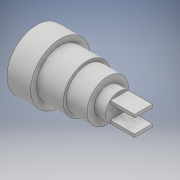
# Autodesk Inventor part: MJ-14
Saved by Autodesk Inventor 2017.3 (Build 213256000, 256)
## iProperties
Part Number: MJ-14
Material: 一般
Document SubType Name: Modeling
Designer: sktom
Density: 1 g/cm^3
Appearance: 既定
Author: sktom
Autodesk Inventor part; units mm, degrees
ref_plane "YZ Plane" through (0, 0, 0) normal (1, 0, 0) x (0, 1, 0)
ref_plane "XZ Plane" through (0, 0, 0) normal (0, 1, 0) x (-1, 0, 0)
ref_plane "XY Plane" through (0, 0, 0) normal (0, 0, 1) x (1, 0, 0)
sketch "スケッチ1" plane through (0, 0, 0) normal (0, 0, 1) x (1, 0, 0)
  line L0 (0, 0) -> (0, 5)
  line L1 (0, 5) -> (4, 5)
  line L2 (4, 5) -> (4, 4)
  line L3 (4, 4) -> (8.5, 4)
  line L4 (8.5, 4) -> (8.5, 3.5)
  line L5 (8.5, 3.5) -> (12, 3.5)
  line L6 (12, 3.5) -> (12, 2.25)
  line L7 (12, 2.25) -> (13.9, 2.25)
  line L8 (13.9, 2.25) -> (13.9, 0)
  line L9 (13.9, 0) -> (0, 0)
  dimension "d0" = 4
  dimension "d1" = 4.5
  dimension "d2" = 8
  dimension "d3" = 1.9
  dimension "d4" = 5
  dimension "d5" = 4
  dimension "d6" = 3.5
  dimension "d7" = 2.25
  constraints: 20 end point, 7 perpendicular, 2 horizontal, 1 vertical
  measures "d0" distance of L0.end L1.end
  measures "d1" distance of L2.end L3.end
  measures "d2" distance between parallel lines of L2 L6
  measures "d3" distance of L6.end L7.end
  measures "d4" distance of L0.start L0.end
  measures "d5" distance between parallel lines of L9 L3
  measures "d6" distance between parallel lines of L9 L5
  measures "d7" distance between parallel lines of L9 L7
revolve "回転1" add sketch "スケッチ1" angle 360 about axis through (13.9, 0, 0) along (-1, 0, 0)
sketch "スケッチ2" plane through (13.9, 0, 0) normal (1, 0, 0) x (0, 0, -1)
  circle A0 centre (0, 0) radius 2.25 projected
  line L0 (-1.6771, 1.5) -> (-1.1771, 1.5)
  line L1 (-1.1771, 1.5) -> (-1.1771, -1.5)
  line L2 (-1.1771, -1.5) -> (-1.6771, -1.5)
  line L3 (-1.6771, -1.5) -> (-1.6771, 1.5)
  line L4 (1.6771, 1.5) -> (1.1771, 1.5)
  line L5 (1.1771, 1.5) -> (1.1771, -1.5)
  line L6 (1.1771, -1.5) -> (1.6771, -1.5)
  line L7 (1.6771, -1.5) -> (1.6771, 1.5)
  point P0 (-1.1771, 0)
  point P1 (1.1771, 0)
  dimension "d9" = 3
  dimension "d10" = 0.5
  constraints: 16 end point, 4 parallel, 2 horizontal, 2 horizontal alignment, 2 midpoint, 2 perpendicular, 2 point on circle, 2 point on line, 1 collinear
  measures "d9" distance of L0.end L1.end
  measures "d10" distance of L0.start L0.end
extrude "押し出し1" add sketch "スケッチ2" along normal blind 4.1 contours L7 L6 L5 L4 | L0 L1 L2 L3
